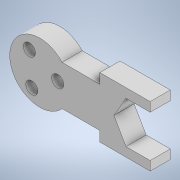
# Autodesk Inventor part: Деталь1
Saved by Autodesk Inventor 2020 (Build 240168000, 168)
## iProperties
Created: 2020-03-28
Part Number: Деталь1
Material: Типовые
Document SubType Name: Modeling
Designer: Trickster2038
Density: 1 g/cm^3
Appearance: По умолчанию
Author: Trickster2038
Autodesk Inventor part; units mm, degrees
ref_plane "YZ Plane" through (0, 0, 0) normal (1, 0, 0) x (0, 1, 0)
ref_plane "XZ Plane" through (0, 0, 0) normal (0, 1, 0) x (-1, 0, 0)
ref_plane "XY Plane" through (0, 0, 0) normal (0, 0, 1) x (1, 0, 0)
sketch "Эскиз1" plane through (0, 0, 0) normal (0, 0, 1) x (1, 0, 0)
  point P0 (0, 0)
sketch "Эскиз2" plane through (0, 0, 0) normal (0, 0, 1) x (1, 0, 0)
  circle A0 centre (0, 0) radius 9
  circle A1 centre (0, 0) radius 14.9355
  line L0 (29.9138, -9.957) -> (11.1323, -9.957)
  line L1 (11.0941, 9.9995) -> (29.9138, 9.9995)
  line L2 (11.0941, 9.9995) -> (29.9138, 9.9995)
  line L3 (29.9138, 9.9995) -> (29.9138, 14.9995)
  line L4 (29.9138, 14.9995) -> (54.9138, 14.9995)
  line L5 (29.9138, -9.957) -> (29.9138, -14.9572)
  line L6 (29.9138, -14.9572) -> (54.9138, -14.9572)
  line L7 (-18.0074, -0.0005) -> (54.9138, -0.0005)
  line L8 (54.9138, 14.9995) -> (48.9138, 14.9995)
  line L9 (48.9138, 14.9995) -> (48.9138, -8.0243)
  line L10 (42.9138, 10.3918) -> (54.9138, 10.3918)
  line L11 (54.9138, -10.3928) -> (42.9138, -10.3928)
  line L12 (42.9138, -10.3928) -> (36.9138, -0.0005)
  line L13 (36.9138, -0.0005) -> (42.9138, 10.3918)
  line L14 (54.9138, 14.9995) -> (54.9138, 10.3918)
  line L15 (54.9138, -14.9572) -> (54.9138, -10.3928)
  line L16 (0, 0) -> (22.1205, 0) construction
  line L17 (0, 0) -> (18.5985, 0) construction
  line L18 (0, 0) -> (18.6696, 0) construction
  line L19 (0, 0) -> (12.4111, 0) construction
  circle A2 centre (-5.1622, 7.3724) radius 3
  circle A3 centre (-3.9303, -8.4286) radius 3
  circle A4 centre (8.9658, 0.7844) radius 3
  point P0 (48.9138, -0.0005)
  point P1 (48.9138, -0.0005)
  point P2 (48.9138, -0.0005)
  constraints: 40 end point, 7 horizontal, 5 centre point, 5 perpendicular, 4 point on circle, 3 coincident, 3 point on line, 2 collinear, 1 parallel, 1 vertical, 8 other
extrude "Выдавливание1" add sketch "Эскиз2" along normal blind 10 contours A4 L7 A0 A2 | A0 A2 L7 A1 A4 | A4 L7 A1 A0 A3 | A0 A3 L7 A4 | L7 L12 L11 L15 L6 L5 L0 A1 | A1 L1 L3 L4 L9 L10 L13 L7 | L9 L4 L14 L10
